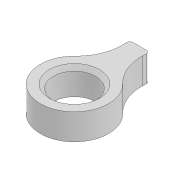
# Autodesk Inventor part: thumb_bolt_converter
Saved by Autodesk Inventor 2020 (Build 240168000, 168)
## iProperties
Created: 2020-07-20
Part Number: thumb_bolt_converter
Material: Generic
Document SubType Name: Modeling
Designer: Daniel
Density: 1 g/cm^3
Appearance: Default
Author: Daniel
Autodesk Inventor part; units mm, degrees
ref_plane "YZ Plane" through (0, 0, 0) normal (1, 0, 0) x (0, 1, 0)
ref_plane "XZ Plane" through (0, 0, 0) normal (0, 1, 0) x (-1, 0, 0)
ref_plane "XY Plane" through (0, 0, 0) normal (0, 0, 1) x (1, 0, 0)
sketch "Sketch1" plane through (0, 0, 0) normal (0, 1, 0) x (-1, 0, 0)
  circle A0 centre (0, 0) radius 3.25
  circle A1 centre (0, 0) radius 5.25
  line L0 (1.5, -5.0312) -> (-1.5, -5.0312)
  line L1 (-1.5, -5.0312) -> (-1.5, -10.0312)
  line L2 (-1.5, -10.0312) -> (1.5, -10.0312)
  line L3 (1.5, -10.0312) -> (1.5, -5.0312)
  line L4 (0, 0) -> (0, -10.0312)
  arc A2 (3.6415, -3.7818) -> (1.5, -9.0312) centre (8.4969, -8.8241) ccw
  arc A3 (-1.5, -9.0312) -> (-3.6415, -3.7818) centre (-8.4969, -8.8241) ccw
  dimension "d0" = 6.5
  dimension "d1" = 2
  dimension "d2" = 1.5
  dimension "d3" = 5
  dimension "d4" = 7
  dimension "d5" = 4
  dimension "d6" = 7
  constraints: 10 end point, 8 point on circle, 4 centre point, 2 parallel, 2 point on line, 2 tangent, 1 coincident, 1 horizontal, 1 horizontal alignment, 1 midpoint, 1 perpendicular
  measures "d0" diameter of A0
  measures "d1" radial gap between concentric circles of A0 A1
  measures "d2" distance between parallel lines of L4 L3
  measures "d3" distance of L2.end L0.start
  measures "d4" radius of A2
  measures "d5" distance of L0.end A3.start
  measures "d6" radius of A3
extrude "Extrusion1" add sketch "Sketch1" along normal blind 4
sketch "Sketch2" plane through (0, 4, 0) normal (0, 1, 0) x (1, 0, 0)
  arc A0 (-3.6415, 3.7818) -> (-1.5, 9.0312) centre (-8.4969, 8.8241) ccw projected
  arc A1 (-3.6415, 3.7818) -> (3.6415, 3.7818) centre (0, 0) ccw projected
  arc A2 (1.5, 9.0312) -> (3.6415, 3.7818) centre (8.4969, 8.8241) ccw projected
  line L0 (1.5, 9.0312) -> (1.5, 10.0312) projected
  line L1 (1.5, 10.0312) -> (-1.5, 10.0312) projected
  line L2 (-1.5, 10.0312) -> (-1.5, 9.0312) projected
  circle A3 centre (0, 0) radius 3.25 projected
  line L3 (-8.6908, -12.2142) -> (10.4061, -12.2142)
  line L4 (10.4061, -12.2142) -> (10.4061, 17.7463)
  line L5 (10.4061, 17.7463) -> (-8.6908, 17.7463)
  line L6 (-8.6908, 17.7463) -> (-8.6908, -12.2142)
  constraints: 8 end point, 2 parallel, 1 horizontal, 1 perpendicular
fillet "Fillet2" radius 0.5 2 edges at (1.5, 2, -10.0312) (-1.5, 2, -10.0312)
chamfer "Chamfer1" distance 0.6 angle 45 1 edges at (3.25, 4, 0)
sketch "Sketch3" plane through (1.5, 0, -9.0312) normal (1, 0, 0) x (0, 0, -1)
  line L0 (-5.2494, 4) -> (0, 4) construction
  line L1 (-2, 6) -> (1, 6)
  line L2 (1, 0) -> (1, 4) construction
  line L3 (1, 6) -> (1, 4)
  line L4 (0, 4) -> (1, 4) construction
  line L5 (-6, 4) -> (-2, 6)
  line L6 (-6, 4) -> (1, 4)
  point P0 (-9.0312, 0)
  dimension "d9" = 2
  dimension "d10" = 7
  dimension "d11" = 3
  constraints: 8 end point, 2 horizontal, 1 collinear, 1 point on line
  measures "d9" distance between parallel lines of L4 L1
  measures "d10" distance of L2.end L5.start
  measures "d11" distance of L1.start L1.end
equation "\"d6\" = d4"
body "Solid1"
